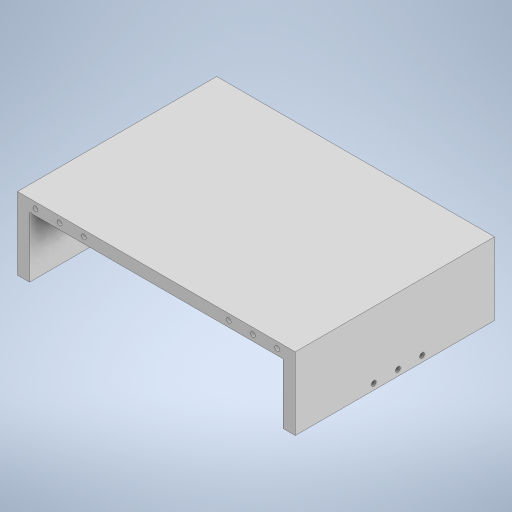
# Autodesk Inventor part: BatteryBoxV2-Top
Saved by Autodesk Inventor 2024 (Build 280153000, 153)
## iProperties
Created: 2025-03-26
Part Number: BatteryBoxV2-Top
Material: Generic
Document SubType Name: Modeling
Designer: v
Density: 1 g/cm^3
Appearance: Default
Author: v
Autodesk Inventor part; units mm, degrees
ref_plane "YZ Plane" through (0, 0, 0) normal (1, 0, 0) x (0, 1, 0)
ref_plane "XZ Plane" through (0, 0, 0) normal (0, 1, 0) x (-1, 0, 0)
ref_plane "XY Plane" through (0, 0, 0) normal (0, 0, 1) x (1, 0, 0)
sketch "TopBoxFrame" plane through (0, 0, 0) normal (0, 0, 1) x (1, 0, 0)
  line L0 (0, 0) -> (292.1, 0)
  line L1 (292.1, 0) -> (292.1, 76.2)
  line L2 (292.1, 76.2) -> (0, 76.2)
  line L3 (0, 76.2) -> (0, 0)
  dimension "d3" = 76.2
  dimension "d27" = 292.1
  constraints: 8 end point, 2 parallel, 1 horizontal, 1 perpendicular
  measures "d3" distance of L0.end L1.end
  measures "d27" distance of L1.end L2.end
extrude "TopBoxWidth" add sketch "TopBoxFrame" against normal blind 209.55
sketch "TrayShape" plane through (0, 0, 0) normal (0, 0, 1) x (1, 0, 0)
  line L0 (12.7, 63.5) -> (279.4, 63.5)
  line L1 (279.4, 63.5) -> (279.4, 0)
  line L2 (279.4, 0) -> (12.7, 0)
  line L3 (12.7, 0) -> (12.7, 63.5)
  line L4 (292.1, 76.2) -> (0, 76.2) projected
  line L5 (0, 76.2) -> (0, 0) projected
  line L6 (292.1, 0) -> (292.1, 76.2) projected
  line L7 (0, 0) -> (292.1, 0) projected
  dimension "d4" = 12.7
  dimension "d5" = 12.7
  dimension "d6" = 12.7
  dimension "d9" = 0
  constraints: 8 end point, 2 parallel, 1 horizontal, 1 perpendicular
  measures "d4" distance between parallel lines of L4 L0
  measures "d5" distance between parallel lines of L5 L3
  measures "d6" distance between parallel lines of L6 L1
  measures "d9" distance between parallel lines of L7 L2
extrude "TrayCut" cut sketch "TrayShape" against normal blind 196.85 contours L0 L1 L2 L3
sketch "HoleGeometry" plane through (0, 0, 0) normal (0, 0, 1) x (1, 0, 0)
  line L0 (292.1, 0) -> (292.1, 76.2) projected
  line L1 (279.4, 63.5) -> (279.4, 0) projected
  line L2 (279.4, 0) -> (292.1, 0) projected
  line L3 (292.1, 0) -> (292.1, 76.2) projected
  line L4 (292.1, 76.2) -> (0, 76.2) projected
  line L5 (0, 76.2) -> (0, 0) projected
  line L6 (0, 0) -> (12.7, 0) projected
  line L7 (12.7, 0) -> (12.7, 63.5) projected
  line L8 (12.7, 63.5) -> (279.4, 63.5) projected
  line L9 (292.1, 76.2) -> (292.1, 0) projected
  line L10 (292.1, 0) -> (0, 0) projected
  line L11 (0, 0) -> (0, 76.2) projected
  line L12 (0, 76.2) -> (292.1, 76.2) projected
  point P0 (273.05, 69.85)
  point P1 (247.65, 69.85)
  point P2 (222.25, 69.85)
  point P3 (69.85, 69.85)
  point P4 (44.45, 69.85)
  point P5 (19.05, 69.85)
  dimension "d35" = 19.05
  dimension "d38" = 25.4
  dimension "d45" = 203.2
  dimension "d108" = 6.35
  constraints: 2 horizontal, 5 other
  measures "d35" distance from line of L0 point (273.05, 69.85)
  measures "d38" distance of point (273.05, 69.85) point (247.65, 69.85)
  measures "d45" distance of point (273.05, 69.85) point (69.85, 69.85)
  measures "d108" distance from line of L4 point (273.05, 69.85)
hole "FrontPlateHoles" at (273.05, 69.85, 0) at (247.65, 69.85, 0) at (222.25, 69.85, 0) at (69.85, 69.85, 0) at (44.45, 69.85, 0) at (19.05, 69.85, 0) direction (0, 0, -1) diameter 5.1054 depth 50.8 tip angle 118 clearance for "Flat Head Machine Screw (82)" size "#10" standard "Ansi Unified Screw Threads"
sketch "BackHoleGeo" plane through (0, 0, -209.55) normal (0, 0, -1) x (-1, 0, 0)
  line L0 (-292.1, 76.2) -> (-292.1, 0) projected
  line L1 (-292.1, 0) -> (0, 0) projected
  line L2 (0, 0) -> (0, 76.2) projected
  line L3 (0, 76.2) -> (-292.1, 76.2) projected
  point P0 (-273.05, 69.85)
  point P1 (-247.65, 69.85)
  point P2 (-222.25, 69.85)
  point P3 (-69.85, 69.85)
  point P4 (-44.45, 69.85)
  point P5 (-19.05, 69.85)
  dimension "d57" = 19.05
  dimension "d60" = 25.4
  dimension "d67" = 203.2
  dimension "d107" = 6.35
  constraints: 2 horizontal, 5 other
  measures "d57" distance from line of L0 point (-273.05, 69.85)
  measures "d60" distance of point (-273.05, 69.85) point (-247.65, 69.85)
  measures "d67" distance of point (-273.05, 69.85) point (-69.85, 69.85)
  measures "d107" distance from line of L3 point (-273.05, 69.85)
hole "BackPlateHoles" at (273.05, 69.85, -209.55) at (247.65, 69.85, -209.55) at (222.25, 69.85, -209.55) at (69.85, 69.85, -209.55) at (44.45, 69.85, -209.55) at (19.05, 69.85, -209.55) direction (0, 0, 1) diameter 5.1054 depth 50.8 tip angle 118 clearance for "Flat Head Machine Screw (82)" size "#10" standard "Ansi Unified Screw Threads"
sketch "RightHoleGeo" plane through (292.1, 0, 0) normal (1, 0, 0) x (0, 0, -1)
  line L0 (0, 76.2) -> (209.55, 76.2) projected
  line L1 (0, 0) -> (0, 76.2) projected
  line L2 (0, 0) -> (209.55, 0) projected
  point P0 (82.55, 6.35)
  point P1 (107.95, 6.35)
  point P2 (133.35, 6.35)
  dimension "d80" = 82.55
  dimension "d83" = 25.4
  dimension "d104" = 6.35
  constraints: 1 horizontal, 2 other
  measures "d80" distance from line of L1 point (82.55, 6.35)
  measures "d83" distance of point (82.55, 6.35) point (107.95, 6.35)
  measures "d104" distance from line of L2 point (82.55, 6.35)
hole "RightPlateHoles" at (292.1, 6.35, -82.55) at (292.1, 6.35, -107.95) at (292.1, 6.35, -133.35) direction (-1, 0, 0) diameter 5.1054 depth 50.8 tip angle 118 clearance for "Flat Head Machine Screw (82)" size "#10" standard "Ansi Unified Screw Threads"
sketch "LeftHoleGeo" plane through (0, 0, 0) normal (-1, 0, 0) x (0, 0, 1)
  line L0 (0, 76.2) -> (-209.55, 76.2) projected
  line L1 (-209.55, 0) -> (-209.55, 76.2) projected
  line L2 (0, 0) -> (-209.55, 0) projected
  point P0 (-127, 6.35)
  point P1 (-101.6, 6.35)
  point P2 (-76.2, 6.35)
  dimension "d96" = 82.55
  dimension "d99" = 25.4
  dimension "d105" = 6.35
  constraints: 1 horizontal, 2 other
  measures "d96" distance from line of L1 point (-127, 6.35)
  measures "d99" distance of point (-127, 6.35) point (-101.6, 6.35)
  measures "d105" distance from line of L2 point (-127, 6.35)
hole "LeftPlateHoles" at (0, 6.35, -127) at (0, 6.35, -101.6) at (0, 6.35, -76.2) direction (1, 0, 0) diameter 5.1054 depth 50.8 tip angle 118 clearance for "Flat Head Machine Screw (82)" size "#10" standard "Ansi Unified Screw Threads"
equation "\"d5\" = d4"
equation "\"d6\" = d5"
body "Solid1"
